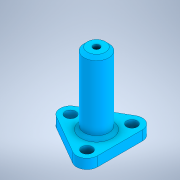
# Autodesk Inventor part: caster-bng
Saved by Autodesk Inventor 2020 (Build 240168000, 168)
## iProperties
Created: 2020-11-05
Part Number: caster-bng
Material: Generic
Document SubType Name: Modeling
Designer: alnwlsn
Density: 1 g/cm^3
Appearance: Default
Author: alnwlsn
Autodesk Inventor part; units mm, degrees
ref_plane "YZ Plane" through (0, 0, 0) normal (1, 0, 0) x (0, 1, 0)
ref_plane "XZ Plane" through (0, 0, 0) normal (0, 1, 0) x (-1, 0, 0)
ref_plane "XY Plane" through (0, 0, 0) normal (0, 0, 1) x (1, 0, 0)
sketch "Sketch1" plane through (0, 0, 0) normal (0, 0, 1) x (1, 0, 0)
  line L0 (0, 0) -> (0, 38.4841) construction
  line L1 (2.8, 25) -> (3.8, 24)
  line L2 (3.8, 24) -> (3.8, 4)
  line L3 (3.8, 4) -> (4.8, 3)
  line L4 (4.8, 3) -> (11.9, 3)
  line L5 (11.9, 3) -> (12, 2.9)
  line L6 (12, 2.9) -> (12, 0)
  line L7 (12, 0) -> (1, 0)
  line L8 (2.8, 25) -> (1, 25)
  line L9 (1, 25) -> (1, 0)
  dimension "d0" = 135
  dimension "d1" = 1
  dimension "d2" = 2.8
  dimension "d3" = 25
  dimension "d4" = 12
  dimension "d5" = 3
  dimension "d6" = 0.1
  dimension "d7" = 1
  dimension "d8" = 1
  constraints: 20 end point, 3 parallel, 2 perpendicular, 1 horizontal, 1 point on line, 1 vertical
  measures "d0" angle of L6 L5
  measures "d1" distance between parallel lines of L0 L9
  measures "d2" distance between parallel lines of L2 L9
  measures "d3" distance between parallel lines of L7 L8
  measures "d4" distance between parallel lines of L0 L6
  measures "d5" distance between parallel lines of L7 L4
  measures "d6" horizontal distance of L5.end L4.end
  measures "d7" horizontal distance of L3.end L2.end
  measures "d8" horizontal distance of L1.end L1.start
revolve "Revolution1" add sketch "Sketch1" angle 360 about axis through (0, 0, 0) along (0, 1, 0)
sketch "Sketch2" plane through (0, 3, 0) normal (0, 1, 0) x (1, 0, 0)
  line L0 (0, 0) -> (-8, 0) construction
  circle A0 centre (-8, 0) radius 1.65
  dimension "d10" = 3.3
  dimension "d11" = 8
  constraints: 2 end point, 1 centre point, 1 coincident, 1 horizontal
  measures "d10" diameter of A0
  measures "d11" distance of L0.start L0.end
extrude "Extrusion1" cut sketch "Sketch2" against normal blind 10
pattern_circular "Circular Pattern1" count 3 over 360 about axis through (0, 14, 0) along (0, -1, 0) of "Extrusion1"
sketch "Sketch3" plane through (0, 3, 0) normal (0, 1, 0) x (1, 0, 0)
  circle A0 centre (4, 6.9282) radius 1.65 projected
  circle A1 centre (4, -6.9282) radius 1.65 projected
  circle A2 centre (-8, 0) radius 1.65 projected
  circle A3 centre (4, 6.9282) radius 3.2
  circle A4 centre (4, -6.9282) radius 3.2
  circle A5 centre (-8, 0) radius 3.2
  line L0 (-9.6, -2.7713) -> (2.4, -9.6995)
  line L1 (2.4, 9.6995) -> (-9.6, 2.7713)
  line L2 (7.2, -6.9282) -> (7.2, 6.9282)
  circle A6 centre (0, 0) radius 1 projected
  circle A7 centre (0, 0) radius 23.7767
  dimension "d17" = 6.4
  constraints: 6 end point, 6 point on circle, 6 tangent, 4 centre point, 2 equal radius, 1 coincident
  measures "d17" diameter of A4
extrude "Extrusion2" cut sketch "Sketch3" against normal through all contours A7
body "Solid1"
